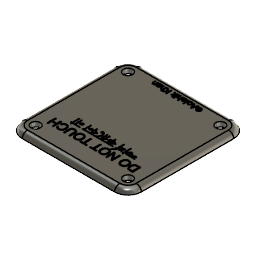
Sensor_Top (Autodesk Fusion 360 design; units mm, degrees)
part number: 2026-02-07-13-48-56-829
Autodesk Fusion 360 part; units mm, degrees
(part 1 of 2)
sketch "Sketch1" plane through (0, 0, 0) normal (0, 0, 1) x (1, 0, 0)
  line L0 (64.1962, 5) -> (20.1962, 5)
  line L1 (20.1962, 5) -> (20.1962, 49)
  line L2 (20.1962, 49) -> (64.1962, 49)
  line L3 (64.1962, 49) -> (64.1962, 5)
  circle A0 centre (59.1962, 10) radius 1.7
  circle A1 centre (25.1962, 10) radius 1.7
  circle A2 centre (59.1962, 44) radius 1.7
  circle A3 centre (25.1962, 44) radius 1.7
  dimension "d1" = 44
  dimension "d2" = 44
  dimension "d3" = 3.4
  dimension "d4" = 3.4
  dimension "d5" = 3.4
  dimension "d6" = 3.4
  dimension "d7" = 5
  dimension "d8" = 5
  dimension "d9" = 5
  dimension "d10" = 5
  dimension "d11" = 5
  dimension "d12" = 5
  dimension "d13" = 5
  dimension "d14" = 5
  constraint horizontal L0
  constraint vertical L1
  constraint horizontal L2
  constraint vertical L3
  measures "d1" distance of L0.start L0.end
  measures "d2" distance of L0.start L2.end
  measures "d3" diameter of A0
  measures "d4" diameter of A1
  measures "d5" diameter of A2
  measures "d6" diameter of A3
  measures "d7" distance of L3 A2.centre
  measures "d8" distance of L2 A2.centre
  measures "d9" distance of L2 A3.centre
  measures "d10" distance of L1 A3.centre
  measures "d11" distance of L1 A1.centre
  measures "d12" distance of L0 A1.centre
  measures "d13" distance of L0 A0.centre
  measures "d14" distance of L3 A0.centre
extrude "Extrude1" add sketch "Sketch1" along normal blind 1.75
sketch "Sketch2" plane through (0, 0, 1.75) normal (0, 0, 1) x (1, 0, 0)
  line L0 (57.9977, 15.8736) -> (57.9932, 12.8736)
  line L1 (57.9932, 12.8736) -> (56.9598, 12.8752)
  spline S0 degree 2 poles (56.9598, 12.8752) (56.6098, 12.8757) (56.4257, 12.9189) knots 0 0 0 1 1 1
  spline S1 degree 2 poles (56.4257, 12.9189) (56.168, 12.9787) (55.9861, 13.1345) knots 0 0 0 1 1 1
  spline S2 degree 2 poles (55.9861, 13.1345) (55.749, 13.3354) (55.6318, 13.6476) knots 0 0 0 1 1 1
  spline S3 degree 2 poles (55.6318, 13.6476) (55.5146, 13.9599) (55.5152, 14.361) knots 0 0 0 1 1 1
  spline S4 degree 2 poles (55.5152, 14.361) (55.5157, 14.7027) (55.5959, 14.9666) knots 0 0 0 1 1 1
  spline S5 degree 2 poles (55.5959, 14.9666) (55.6761, 15.2304) (55.8012, 15.4032) knots 0 0 0 1 1 1
  spline S6 degree 2 poles (55.8012, 15.4032) (55.9263, 15.5759) (56.0748, 15.6749) knots 0 0 0 1 1 1
  spline S7 degree 2 poles (56.0748, 15.6749) (56.2233, 15.7739) (56.4332, 15.8248) knots 0 0 0 1 1 1
  spline S8 degree 2 poles (56.4332, 15.8248) (56.643, 15.8756) (56.9152, 15.8752) knots 0 0 0 1 1 1
  line L2 (56.9152, 15.8752) -> (57.9977, 15.8736)
  line L3 (57.6002, 15.5202) -> (56.9596, 15.5211)
  spline S9 degree 2 poles (56.9596, 15.5211) (56.6629, 15.5216) (56.494, 15.4666) knots 0 0 0 1 1 1
  spline S10 degree 2 poles (56.494, 15.4666) (56.3251, 15.4116) (56.2247, 15.3115) knots 0 0 0 1 1 1
  spline S11 degree 2 poles (56.2247, 15.3115) (56.0833, 15.1705) (56.0041, 14.9322) knots 0 0 0 1 1 1
  spline S12 degree 2 poles (56.0041, 14.9322) (55.925, 14.6939) (55.9245, 14.3542) knots 0 0 0 1 1 1
  spline S13 degree 2 poles (55.9245, 14.3542) (55.9238, 13.8835) (56.0779, 13.6306) knots 0 0 0 1 1 1
  spline S14 degree 2 poles (56.0779, 13.6306) (56.232, 13.3776) (56.4529, 13.2913) knots 0 0 0 1 1 1
  spline S15 degree 2 poles (56.4529, 13.2913) (56.6124, 13.2297) (56.9664, 13.2292) knots 0 0 0 1 1 1
  line L4 (56.9664, 13.2292) -> (57.5967, 13.2282)
  line L5 (57.5967, 13.2282) -> (57.6002, 15.5202)
  spline S16 degree 2 poles (55.0896, 14.4168) (55.0885, 13.6699) (54.6868, 13.2479) knots 0 0 0 1 1 1
  spline S17 degree 2 poles (54.6868, 13.2479) (54.2851, 12.826) (53.6507, 12.8269) knots 0 0 0 1 1 1
  spline S18 degree 2 poles (53.6507, 12.8269) (53.2353, 12.8275) (52.902, 13.0265) knots 0 0 0 1 1 1
  spline S19 degree 2 poles (52.902, 13.0265) (52.5687, 13.2255) (52.3943, 13.5808) knots 0 0 0 1 1 1
  spline S20 degree 2 poles (52.3943, 13.5808) (52.2199, 13.9362) (52.2206, 14.3864) knots 0 0 0 1 1 1
  spline S21 degree 2 poles (52.2206, 14.3864) (52.2212, 14.8427) (52.406, 15.2026) knots 0 0 0 1 1 1
  spline S22 degree 2 poles (52.406, 15.2026) (52.5907, 15.5625) (52.9286, 15.7472) knots 0 0 0 1 1 1
  spline S23 degree 2 poles (52.9286, 15.7472) (53.2665, 15.9319) (53.6574, 15.9313) knots 0 0 0 1 1 1
  spline S24 degree 2 poles (53.6574, 15.9313) (54.081, 15.9306) (54.4142, 15.7255) knots 0 0 0 1 1 1
  spline S25 degree 2 poles (54.4142, 15.7255) (54.7475, 15.5204) (54.9189, 15.1661) knots 0 0 0 1 1 1
  spline S26 degree 2 poles (54.9189, 15.1661) (55.0902, 14.8118) (55.0896, 14.4168) knots 0 0 0 1 1 1
  spline S27 degree 2 poles (54.6804, 14.4236) (54.6812, 14.9659) (54.39, 15.2784) knots 0 0 0 1 1 1
  spline S28 degree 2 poles (54.39, 15.2784) (54.0989, 15.5909) (53.6589, 15.5916) knots 0 0 0 1 1 1
  spline S29 degree 2 poles (53.6589, 15.5916) (53.2108, 15.5922) (52.9207, 15.2775) knots 0 0 0 1 1 1
  spline S30 degree 2 poles (52.9207, 15.2775) (52.6307, 14.9628) (52.6298, 14.3837) knots 0 0 0 1 1 1
  spline S31 degree 2 poles (52.6298, 14.3837) (52.6293, 14.0174) (52.7527, 13.744) knots 0 0 0 1 1 1
  spline S32 degree 2 poles (52.7527, 13.744) (52.8761, 13.4706) (53.1143, 13.3199) knots 0 0 0 1 1 1
  spline S33 degree 2 poles (53.1143, 13.3199) (53.3524, 13.1691) (53.6492, 13.1687) knots 0 0 0 1 1 1
  spline S34 degree 2 poles (53.6492, 13.1687) (54.0707, 13.168) (54.375, 13.4571) knots 0 0 0 1 1 1
  spline S35 degree 2 poles (54.375, 13.4571) (54.6794, 13.7462) (54.6804, 14.4236) knots 0 0 0 1 1 1
  line L6 (50.5509, 15.8848) -> (50.5464, 12.8848)
  line L7 (50.5464, 12.8848) -> (50.1392, 12.8854)
  line L8 (50.1392, 12.8854) -> (48.567, 15.2431)
  line L9 (48.567, 15.2431) -> (48.5635, 12.8878)
  line L10 (48.5635, 12.8878) -> (48.1828, 12.8883)
  line L11 (48.1828, 12.8883) -> (48.1873, 15.8883)
  line L12 (48.1873, 15.8883) -> (48.5946, 15.8877)
  line L13 (48.5946, 15.8877) -> (50.1667, 13.5279)
  line L14 (50.1667, 13.5279) -> (50.1703, 15.8853)
  line L15 (50.1703, 15.8853) -> (50.5509, 15.8848)
  spline S36 degree 2 poles (47.6388, 14.428) (47.6376, 13.6811) (47.2359, 13.2591) knots 0 0 0 1 1 1
  spline S37 degree 2 poles (47.2359, 13.2591) (46.8342, 12.8371) (46.1998, 12.8381) knots 0 0 0 1 1 1
  spline S38 degree 2 poles (46.1998, 12.8381) (45.7844, 12.8387) (45.4511, 13.0377) knots 0 0 0 1 1 1
  spline S39 degree 2 poles (45.4511, 13.0377) (45.1179, 13.2367) (44.9434, 13.592) knots 0 0 0 1 1 1
  spline S40 degree 2 poles (44.9434, 13.592) (44.769, 13.9473) (44.7697, 14.3975) knots 0 0 0 1 1 1
  spline S41 degree 2 poles (44.7697, 14.3975) (44.7704, 14.8539) (44.9551, 15.2138) knots 0 0 0 1 1 1
  spline S42 degree 2 poles (44.9551, 15.2138) (45.1398, 15.5737) (45.4777, 15.7583) knots 0 0 0 1 1 1
  spline S43 degree 2 poles (45.4777, 15.7583) (45.8157, 15.943) (46.2065, 15.9425) knots 0 0 0 1 1 1
  spline S44 degree 2 poles (46.2065, 15.9425) (46.6301, 15.9418) (46.9634, 15.7367) knots 0 0 0 1 1 1
  spline S45 degree 2 poles (46.9634, 15.7367) (47.2966, 15.5315) (47.468, 15.1773) knots 0 0 0 1 1 1
  spline S46 degree 2 poles (47.468, 15.1773) (47.6394, 14.823) (47.6388, 14.428) knots 0 0 0 1 1 1
  spline S47 degree 2 poles (47.2295, 14.4348) (47.2303, 14.9771) (46.9392, 15.2896) knots 0 0 0 1 1 1
  spline S48 degree 2 poles (46.9392, 15.2896) (46.648, 15.6021) (46.2081, 15.6027) knots 0 0 0 1 1 1
  spline S49 degree 2 poles (46.2081, 15.6027) (45.7599, 15.6034) (45.4699, 15.2887) knots 0 0 0 1 1 1
  spline S50 degree 2 poles (45.4699, 15.2887) (45.1798, 14.974) (45.179, 14.3949) knots 0 0 0 1 1 1
  spline S51 degree 2 poles (45.179, 14.3949) (45.1784, 14.0286) (45.3018, 13.7552) knots 0 0 0 1 1 1
  spline S52 degree 2 poles (45.3018, 13.7552) (45.4252, 13.4818) (45.6634, 13.3311) knots 0 0 0 1 1 1
  spline S53 degree 2 poles (45.6634, 13.3311) (45.9016, 13.1803) (46.1983, 13.1798) knots 0 0 0 1 1 1
  spline S54 degree 2 poles (46.1983, 13.1798) (46.6198, 13.1792) (46.9242, 13.4683) knots 0 0 0 1 1 1
  spline S55 degree 2 poles (46.9242, 13.4683) (47.2285, 13.7574) (47.2295, 14.4348) knots 0 0 0 1 1 1
  line L16 (43.497, 15.8954) -> (43.4931, 13.2494)
  line L17 (43.4931, 13.2494) -> (44.4815, 13.2479)
  line L18 (44.4815, 13.2479) -> (44.4809, 12.8939)
  line L19 (44.4809, 12.8939) -> (42.103, 12.8974)
  line L20 (42.103, 12.8974) -> (42.1036, 13.2515)
  line L21 (42.1036, 13.2515) -> (43.0961, 13.25)
  line L22 (43.0961, 13.25) -> (43.1, 15.896)
  line L23 (43.1, 15.896) -> (43.497, 15.8954)
  line L24 (39.924, 15.9007) -> (39.9201, 13.2547)
  line L25 (39.9201, 13.2547) -> (40.9085, 13.2533)
  line L26 (40.9085, 13.2533) -> (40.9079, 12.8992)
  line L27 (40.9079, 12.8992) -> (38.53, 12.9028)
  line L28 (38.53, 12.9028) -> (38.5306, 13.2568)
  line L29 (38.5306, 13.2568) -> (39.5231, 13.2553)
  line L30 (39.5231, 13.2553) -> (39.527, 15.9013)
  line L31 (39.527, 15.9013) -> (39.924, 15.9007)
  spline S56 degree 2 poles (38.3216, 14.442) (38.3205, 13.6951) (37.9187, 13.2731) knots 0 0 0 1 1 1
  spline S57 degree 2 poles (37.9187, 13.2731) (37.517, 12.8511) (36.8826, 12.8521) knots 0 0 0 1 1 1
  spline S58 degree 2 poles (36.8826, 12.8521) (36.4672, 12.8527) (36.134, 13.0517) knots 0 0 0 1 1 1
  spline S59 degree 2 poles (36.134, 13.0517) (35.8007, 13.2507) (35.6263, 13.606) knots 0 0 0 1 1 1
  spline S60 degree 2 poles (35.6263, 13.606) (35.4518, 13.9613) (35.4525, 14.4115) knots 0 0 0 1 1 1
  spline S61 degree 2 poles (35.4525, 14.4115) (35.4532, 14.8679) (35.6379, 15.2277) knots 0 0 0 1 1 1
  spline S62 degree 2 poles (35.6379, 15.2277) (35.8226, 15.5876) (36.1605, 15.7723) knots 0 0 0 1 1 1
  spline S63 degree 2 poles (36.1605, 15.7723) (36.4985, 15.957) (36.8893, 15.9564) knots 0 0 0 1 1 1
  spline S64 degree 2 poles (36.8893, 15.9564) (37.3129, 15.9558) (37.6462, 15.7507) knots 0 0 0 1 1 1
  spline S65 degree 2 poles (37.6462, 15.7507) (37.9794, 15.5455) (38.1508, 15.1912) knots 0 0 0 1 1 1
  spline S66 degree 2 poles (38.1508, 15.1912) (38.3222, 14.837) (38.3216, 14.442) knots 0 0 0 1 1 1
  spline S67 degree 2 poles (37.9123, 14.4488) (37.9131, 14.991) (37.622, 15.3036) knots 0 0 0 1 1 1
  spline S68 degree 2 poles (37.622, 15.3036) (37.3308, 15.6161) (36.8909, 15.6167) knots 0 0 0 1 1 1
  spline S69 degree 2 poles (36.8909, 15.6167) (36.4427, 15.6174) (36.1527, 15.3027) knots 0 0 0 1 1 1
  spline S70 degree 2 poles (36.1527, 15.3027) (35.8626, 14.988) (35.8618, 14.4089) knots 0 0 0 1 1 1
  spline S71 degree 2 poles (35.8618, 14.4089) (35.8612, 14.0426) (35.9846, 13.7692) knots 0 0 0 1 1 1
  spline S72 degree 2 poles (35.9846, 13.7692) (36.108, 13.4958) (36.3462, 13.345) knots 0 0 0 1 1 1
  spline S73 degree 2 poles (36.3462, 13.345) (36.5844, 13.1943) (36.8811, 13.1938) knots 0 0 0 1 1 1
  spline S74 degree 2 poles (36.8811, 13.1938) (37.3027, 13.1932) (37.607, 13.4823) knots 0 0 0 1 1 1
  spline S75 degree 2 poles (37.607, 13.4823) (37.9113, 13.7714) (37.9123, 14.4488) knots 0 0 0 1 1 1
  line L32 (32.97, 12.9111) -> (32.573, 12.9117)
  line L33 (32.573, 12.9117) -> (32.5756, 14.645)
  spline S76 degree 2 poles (32.5756, 14.645) (32.5763, 15.0973) (32.679, 15.3632) knots 0 0 0 1 1 1
  spline S77 degree 2 poles (32.679, 15.3632) (32.7817, 15.629) (33.049, 15.7954) knots 0 0 0 1 1 1
  spline S78 degree 2 poles (33.049, 15.7954) (33.3164, 15.9618) (33.7502, 15.9611) knots 0 0 0 1 1 1
  spline S79 degree 2 poles (33.7502, 15.9611) (34.1717, 15.9605) (34.4396, 15.8148) knots 0 0 0 1 1 1
  spline S80 degree 2 poles (34.4396, 15.8148) (34.7075, 15.6691) (34.8216, 15.3937) knots 0 0 0 1 1 1
  spline S81 degree 2 poles (34.8216, 15.3937) (34.9358, 15.1183) (34.9351, 14.6415) knots 0 0 0 1 1 1
  line L34 (34.9351, 14.6415) -> (34.9325, 12.9082)
  line L35 (34.9325, 12.9082) -> (34.5355, 12.9088)
  line L36 (34.5355, 12.9088) -> (34.5381, 14.64)
  spline S82 degree 2 poles (34.5381, 14.64) (34.5387, 15.0309) (34.4663, 15.2162) knots 0 0 0 1 1 1
  spline S83 degree 2 poles (34.4663, 15.2162) (34.394, 15.4015) (34.2171, 15.502) knots 0 0 0 1 1 1
  spline S84 degree 2 poles (34.2171, 15.502) (34.0402, 15.6026) (33.7844, 15.603) knots 0 0 0 1 1 1
  spline S85 degree 2 poles (33.7844, 15.603) (33.3465, 15.6036) (33.16, 15.4054) knots 0 0 0 1 1 1
  spline S86 degree 2 poles (33.16, 15.4054) (32.9735, 15.2072) (32.9726, 14.6424) knots 0 0 0 1 1 1
  line L37 (32.9726, 14.6424) -> (32.97, 12.9111)
  line L38 (29.7745, 14.8641) -> (29.3776, 14.965)
  spline S87 degree 2 poles (29.3776, 14.965) (29.5032, 15.4539) (29.8279, 15.7102) knots 0 0 0 1 1 1
  spline S88 degree 2 poles (29.8279, 15.7102) (30.1526, 15.9665) (30.6213, 15.9658) knots 0 0 0 1 1 1
  spline S89 degree 2 poles (30.6213, 15.9658) (31.1063, 15.9651) (31.4099, 15.7672) knots 0 0 0 1 1 1
  spline S90 degree 2 poles (31.4099, 15.7672) (31.7134, 15.5692) (31.8715, 15.1945) knots 0 0 0 1 1 1
  spline S91 degree 2 poles (31.8715, 15.1945) (32.0295, 14.8198) (32.0289, 14.3901) knots 0 0 0 1 1 1
  spline S92 degree 2 poles (32.0289, 14.3901) (32.0282, 13.9214) (31.8486, 13.5728) knots 0 0 0 1 1 1
  spline S93 degree 2 poles (31.8486, 13.5728) (31.669, 13.2242) (31.3382, 13.0435) knots 0 0 0 1 1 1
  spline S94 degree 2 poles (31.3382, 13.0435) (31.0075, 12.8629) (30.6105, 12.8635) knots 0 0 0 1 1 1
  spline S95 degree 2 poles (30.6105, 12.8635) (30.1603, 12.8642) (29.8537, 13.0939) knots 0 0 0 1 1 1
  spline S96 degree 2 poles (29.8537, 13.0939) (29.547, 13.3235) (29.4269, 13.7391) knots 0 0 0 1 1 1
  line L39 (29.4269, 13.7391) -> (29.8179, 13.8306)
  spline S97 degree 2 poles (29.8179, 13.8306) (29.9218, 13.503) (30.1201, 13.3534) knots 0 0 0 1 1 1
  spline S98 degree 2 poles (30.1201, 13.3534) (30.3183, 13.2037) (30.6192, 13.2032) knots 0 0 0 1 1 1
  spline S99 degree 2 poles (30.6192, 13.2032) (30.965, 13.2027) (31.1975, 13.3681) knots 0 0 0 1 1 1
  spline S100 degree 2 poles (31.1975, 13.3681) (31.43, 13.5335) (31.5246, 13.8127) knots 0 0 0 1 1 1
  spline S101 degree 2 poles (31.5246, 13.8127) (31.6191, 14.0919) (31.6196, 14.3886) knots 0 0 0 1 1 1
  spline S102 degree 2 poles (31.6196, 14.3886) (31.6202, 14.7713) (31.5091, 15.0569) knots 0 0 0 1 1 1
  spline S103 degree 2 poles (31.5091, 15.0569) (31.398, 15.3426) (31.1628, 15.4841) knots 0 0 0 1 1 1
  spline S104 degree 2 poles (31.1628, 15.4841) (30.9277, 15.6257) (30.6535, 15.6261) knots 0 0 0 1 1 1
  spline S105 degree 2 poles (30.6535, 15.6261) (30.3199, 15.6266) (30.0884, 15.4346) knots 0 0 0 1 1 1
  spline S106 degree 2 poles (30.0884, 15.4346) (29.8569, 15.2426) (29.7745, 14.8641) knots 0 0 0 1 1 1
  line L40 (28.8777, 15.9173) -> (28.8732, 12.9173)
  line L41 (28.8732, 12.9173) -> (28.4762, 12.9179)
  line L42 (28.4762, 12.9179) -> (28.478, 14.1498)
  line L43 (28.478, 14.1498) -> (26.9187, 14.1522)
  line L44 (26.9187, 14.1522) -> (26.9168, 12.9202)
  line L45 (26.9168, 12.9202) -> (26.5198, 12.9208)
  line L46 (26.5198, 12.9208) -> (26.5243, 15.9208)
  line L47 (26.5243, 15.9208) -> (26.9213, 15.9202)
  line L48 (26.9213, 15.9202) -> (26.9192, 14.5062)
  line L49 (26.9192, 14.5062) -> (28.4786, 14.5038)
  line L50 (28.4786, 14.5038) -> (28.4807, 15.9179)
  line L51 (28.4807, 15.9179) -> (28.8777, 15.9173)
  line L52 (49.5473, 17.5944) -> (50.0835, 17.5936)
  line L53 (50.0835, 17.5936) -> (50.0876, 20.3111)
  line L54 (50.0876, 20.3111) -> (50.2965, 20.1068)
  line L55 (50.2965, 20.1068) -> (50.2942, 18.6003)
  spline S107 degree 2 poles (50.2942, 18.6003) (50.2941, 18.5506) (50.3137, 18.4878) knots 0 0 0 1 1 1
  spline S108 degree 2 poles (50.3137, 18.4878) (50.3332, 18.425) (50.3645, 18.3634) knots 0 0 0 1 1 1
  spline S109 degree 2 poles (50.3645, 18.3634) (50.3958, 18.3019) (50.431, 18.2456) knots 0 0 0 1 1 1
  spline S110 degree 2 poles (50.431, 18.2456) (50.4662, 18.1894) (50.4975, 18.1501) knots 0 0 0 1 1 1
  line L56 (50.4975, 18.1501) -> (51.5662, 19.1738)
  line L57 (51.5662, 19.1738) -> (51.8798, 19.0059)
  spline S111 degree 2 poles (51.8798, 19.0059) (51.6493, 18.7865) (51.5393, 18.6703) knots 0 0 0 1 1 1
  spline S112 degree 2 poles (51.5393, 18.6703) (51.4293, 18.5541) (51.4292, 18.5148) knots 0 0 0 1 1 1
  spline S113 degree 2 poles (51.4292, 18.5148) (51.4291, 18.4259) (51.497, 18.3761) knots 0 0 0 1 1 1
  spline S114 degree 2 poles (51.497, 18.3761) (51.5649, 18.3263) (51.6539, 18.3262) knots 0 0 0 1 1 1
  spline S115 degree 2 poles (51.6539, 18.3262) (51.7428, 18.3261) (51.8292, 18.3586) knots 0 0 0 1 1 1
  spline S116 degree 2 poles (51.8292, 18.3586) (51.9155, 18.3912) (52.0032, 18.4303) knots 0 0 0 1 1 1
  spline S117 degree 2 poles (52.0032, 18.4303) (52.0909, 18.4694) (52.1786, 18.5019) knots 0 0 0 1 1 1
  spline S118 degree 2 poles (52.1786, 18.5019) (52.2662, 18.5345) (52.3578, 18.5344) knots 0 0 0 1 1 1
  spline S119 degree 2 poles (52.3578, 18.5344) (52.4912, 18.5342) (52.6048, 18.4791) knots 0 0 0 1 1 1
  spline S120 degree 2 poles (52.6048, 18.4791) (52.7185, 18.424) (52.8073, 18.331) knots 0 0 0 1 1 1
  spline S121 degree 2 poles (52.8073, 18.331) (52.8961, 18.238) (52.9587, 18.1189) knots 0 0 0 1 1 1
  spline S122 degree 2 poles (52.9587, 18.1189) (53.0213, 17.9998) (53.0499, 17.8742) knots 0 0 0 1 1 1
  spline S123 degree 2 poles (53.0499, 17.8742) (53.1626, 18.0519) (53.2374, 18.1943) knots 0 0 0 1 1 1
  spline S124 degree 2 poles (53.2374, 18.1943) (53.3121, 18.3368) (53.3672, 18.4361) knots 0 0 0 1 1 1
  spline S125 degree 2 poles (53.3672, 18.4361) (53.4223, 18.5354) (53.4681, 18.5876) knots 0 0 0 1 1 1
  spline S126 degree 2 poles (53.4681, 18.5876) (53.514, 18.6399) (53.5689, 18.6398) knots 0 0 0 1 1 1
  spline S127 degree 2 poles (53.5689, 18.6398) (53.6108, 18.6397) (53.6656, 18.6161) knots 0 0 0 1 1 1
  spline S128 degree 2 poles (53.6656, 18.6161) (53.7205, 18.5925) (53.7845, 18.5374) knots 0 0 0 1 1 1
  spline S129 degree 2 poles (53.7845, 18.5374) (53.8485, 18.4824) (53.9203, 18.3908) knots 0 0 0 1 1 1
  spline S130 degree 2 poles (53.9203, 18.3908) (53.9921, 18.2991) (54.0678, 18.163) knots 0 0 0 1 1 1
  line L58 (54.0678, 18.163) -> (53.9395, 18.0821)
  spline S131 degree 2 poles (53.9395, 18.0821) (53.9212, 18.1214) (53.8964, 18.1619) knots 0 0 0 1 1 1
  spline S132 degree 2 poles (53.8964, 18.1619) (53.8717, 18.2025) (53.8429, 18.2353) knots 0 0 0 1 1 1
  spline S133 degree 2 poles (53.8429, 18.2353) (53.8142, 18.268) (53.7855, 18.2903) knots 0 0 0 1 1 1
  spline S134 degree 2 poles (53.7855, 18.2903) (53.7567, 18.3126) (53.7306, 18.3126) knots 0 0 0 1 1 1
  spline S135 degree 2 poles (53.7306, 18.3126) (53.6573, 18.3127) (53.6075, 18.2448) knots 0 0 0 1 1 1
  spline S136 degree 2 poles (53.6075, 18.2448) (53.5577, 18.1768) (53.5053, 18.071) knots 0 0 0 1 1 1
  spline S137 degree 2 poles (53.5053, 18.071) (53.4528, 17.9651) (53.3833, 17.8371) knots 0 0 0 1 1 1
  spline S138 degree 2 poles (53.3833, 17.8371) (53.3138, 17.709) (53.1985, 17.5889) knots 0 0 0 1 1 1
  line L59 (53.1985, 17.5889) -> (54.1323, 17.5875)
  line L60 (54.1323, 17.5875) -> (54.2758, 17.3911)
  line L61 (54.2758, 17.3911) -> (52.1573, 17.3943)
  line L62 (52.1573, 17.3943) -> (52.0242, 17.5907)
  line L63 (52.0242, 17.5907) -> (52.0059, 17.6221)
  spline S139 degree 2 poles (52.0059, 17.6221) (51.8776, 17.5229) (51.7232, 17.4617) knots 0 0 0 1 1 1
  spline S140 degree 2 poles (51.7232, 17.4617) (51.5688, 17.4004) (51.3962, 17.4007) knots 0 0 0 1 1 1
  spline S141 degree 2 poles (51.3962, 17.4007) (51.1948, 17.401) (51.0314, 17.4588) knots 0 0 0 1 1 1
  spline S142 degree 2 poles (51.0314, 17.4588) (50.868, 17.5166) (50.7348, 17.6175) knots 0 0 0 1 1 1
  spline S143 degree 2 poles (50.7348, 17.6175) (50.6015, 17.7184) (50.4932, 17.8545) knots 0 0 0 1 1 1
  spline S144 degree 2 poles (50.4932, 17.8545) (50.3848, 17.9907) (50.2935, 18.1478) knots 0 0 0 1 1 1
  line L64 (50.2935, 18.1478) -> (50.2916, 16.8871)
  spline S145 degree 2 poles (50.2916, 16.8871) (50.242, 16.9107) (50.2094, 16.9761) knots 0 0 0 1 1 1
  spline S146 degree 2 poles (50.2094, 16.9761) (50.1768, 17.0416) (50.1547, 17.1201) knots 0 0 0 1 1 1
  spline S147 degree 2 poles (50.1547, 17.1201) (50.1326, 17.1986) (50.117, 17.2745) knots 0 0 0 1 1 1
  spline S148 degree 2 poles (50.117, 17.2745) (50.1014, 17.3503) (50.0858, 17.3974) knots 0 0 0 1 1 1
  line L65 (50.0858, 17.3974) -> (49.6908, 17.398)
  line L66 (49.6908, 17.398) -> (49.5473, 17.5944)
  spline S149 degree 2 poles (52.09, 17.8914) (52.0899, 17.8103) (52.1225, 17.7475) knots 0 0 0 1 1 1
  spline S150 degree 2 poles (52.1225, 17.7475) (52.1551, 17.6846) (52.2229, 17.5904) knots 0 0 0 1 1 1
  line L67 (52.2229, 17.5904) -> (52.903, 17.5893)
  spline S151 degree 2 poles (52.903, 17.5893) (52.9448, 17.5893) (52.954, 17.6298) knots 0 0 0 1 1 1
  spline S152 degree 2 poles (52.954, 17.6298) (52.9633, 17.6703) (52.9633, 17.7148) knots 0 0 0 1 1 1
  spline S153 degree 2 poles (52.9633, 17.7148) (52.9635, 17.7985) (52.9165, 17.8901) knots 0 0 0 1 1 1
  spline S154 degree 2 poles (52.9165, 17.8901) (52.8696, 17.9817) (52.7925, 18.0577) knots 0 0 0 1 1 1
  spline S155 degree 2 poles (52.7925, 18.0577) (52.7155, 18.1337) (52.6149, 18.1835) knots 0 0 0 1 1 1
  spline S156 degree 2 poles (52.6149, 18.1835) (52.5142, 18.2333) (52.407, 18.2335) knots 0 0 0 1 1 1
  spline S157 degree 2 poles (52.407, 18.2335) (52.3442, 18.2336) (52.2867, 18.2102) knots 0 0 0 1 1 1
  spline S158 degree 2 poles (52.2867, 18.2102) (52.2291, 18.1867) (52.1859, 18.141) knots 0 0 0 1 1 1
  spline S159 degree 2 poles (52.1859, 18.141) (52.1426, 18.0953) (52.1164, 18.0326) knots 0 0 0 1 1 1
  spline S160 degree 2 poles (52.1164, 18.0326) (52.0901, 17.9698) (52.09, 17.8914) knots 0 0 0 1 1 1
  spline S161 degree 2 poles (50.7482, 17.8829) (50.8736, 17.7833) (51.0226, 17.7334) knots 0 0 0 1 1 1
  spline S162 degree 2 poles (51.0226, 17.7334) (51.1716, 17.6835) (51.3286, 17.6833) knots 0 0 0 1 1 1
  spline S163 degree 2 poles (51.3286, 17.6833) (51.4724, 17.683) (51.619, 17.7391) knots 0 0 0 1 1 1
  spline S164 degree 2 poles (51.619, 17.7391) (51.7655, 17.7951) (51.8913, 17.9466) knots 0 0 0 1 1 1
  spline S165 degree 2 poles (51.8913, 17.9466) (51.8861, 17.9754) (51.8836, 18.0041) knots 0 0 0 1 1 1
  spline S166 degree 2 poles (51.8836, 18.0041) (51.881, 18.0329) (51.881, 18.0591) knots 0 0 0 1 1 1
  spline S167 degree 2 poles (51.881, 18.0591) (51.881, 18.0748) (51.8824, 18.0918) knots 0 0 0 1 1 1
  spline S168 degree 2 poles (51.8824, 18.0918) (51.8837, 18.1088) (51.8864, 18.1244) knots 0 0 0 1 1 1
  spline S169 degree 2 poles (51.8864, 18.1244) (51.8392, 18.1088) (51.7895, 18.0971) knots 0 0 0 1 1 1
  spline S170 degree 2 poles (51.7895, 18.0971) (51.7398, 18.0854) (51.6875, 18.0855) knots 0 0 0 1 1 1
  spline S171 degree 2 poles (51.6875, 18.0855) (51.562, 18.0857) (51.4562, 18.1643) knots 0 0 0 1 1 1
  spline S172 degree 2 poles (51.4562, 18.1643) (51.3503, 18.243) (51.2904, 18.4078) knots 0 0 0 1 1 1
  line L68 (51.2904, 18.4078) -> (50.7482, 17.8829)
  line L69 (46.9527, 17.5983) -> (47.4889, 17.5975)
  line L70 (47.4889, 17.5975) -> (47.493, 20.3046)
  line L71 (47.493, 20.3046) -> (47.7019, 20.095)
  line L72 (47.7019, 20.095) -> (47.6993, 18.4028)
  spline S173 degree 2 poles (47.6993, 18.4028) (47.6993, 18.374) (47.7214, 18.3125) knots 0 0 0 1 1 1
  spline S174 degree 2 poles (47.7214, 18.3125) (47.7436, 18.251) (47.7827, 18.1764) knots 0 0 0 1 1 1
  spline S175 degree 2 poles (47.7827, 18.1764) (47.8218, 18.1018) (47.8753, 18.0206) knots 0 0 0 1 1 1
  spline S176 degree 2 poles (47.8753, 18.0206) (47.9288, 17.9395) (47.9888, 17.874) knots 0 0 0 1 1 1
  spline S177 degree 2 poles (47.9888, 17.874) (48.0489, 17.8085) (48.1168, 17.7653) knots 0 0 0 1 1 1
  spline S178 degree 2 poles (48.1168, 17.7653) (48.1848, 17.722) (48.2502, 17.7219) knots 0 0 0 1 1 1
  spline S179 degree 2 poles (48.2502, 17.7219) (48.3077, 17.7218) (48.3522, 17.7453) knots 0 0 0 1 1 1
  spline S180 degree 2 poles (48.3522, 17.7453) (48.3967, 17.7688) (48.4321, 17.8053) knots 0 0 0 1 1 1
  spline S181 degree 2 poles (48.4321, 17.8053) (48.4674, 17.8419) (48.4976, 17.8902) knots 0 0 0 1 1 1
  spline S182 degree 2 poles (48.4976, 17.8902) (48.5277, 17.9386) (48.5566, 17.9882) knots 0 0 0 1 1 1
  spline S183 degree 2 poles (48.5566, 17.9882) (48.3267, 18.1612) (48.2066, 18.334) knots 0 0 0 1 1 1
  spline S184 degree 2 poles (48.2066, 18.334) (48.0866, 18.5068) (48.0868, 18.6481) knots 0 0 0 1 1 1
  spline S185 degree 2 poles (48.0868, 18.6481) (48.087, 18.7657) (48.1577, 18.8402) knots 0 0 0 1 1 1
  spline S186 degree 2 poles (48.1577, 18.8402) (48.2284, 18.9146) (48.3383, 18.9145) knots 0 0 0 1 1 1
  spline S187 degree 2 poles (48.3383, 18.9145) (48.4063, 18.9144) (48.4716, 18.8868) knots 0 0 0 1 1 1
  spline S188 degree 2 poles (48.4716, 18.8868) (48.537, 18.8592) (48.5918, 18.8134) knots 0 0 0 1 1 1
  spline S189 degree 2 poles (48.5918, 18.8134) (48.6467, 18.7675) (48.6845, 18.7073) knots 0 0 0 1 1 1
  spline S190 degree 2 poles (48.6845, 18.7073) (48.7224, 18.6471) (48.7353, 18.5817) knots 0 0 0 1 1 1
  spline S191 degree 2 poles (48.7353, 18.5817) (48.7694, 18.6444) (48.8166, 18.7071) knots 0 0 0 1 1 1
  spline S192 degree 2 poles (48.8166, 18.7071) (48.8638, 18.7698) (48.9201, 18.8207) knots 0 0 0 1 1 1
  spline S193 degree 2 poles (48.9201, 18.8207) (48.9764, 18.8716) (49.0379, 18.9029) knots 0 0 0 1 1 1
  spline S194 degree 2 poles (49.0379, 18.9029) (49.0994, 18.9342) (49.1622, 18.9341) knots 0 0 0 1 1 1
  spline S195 degree 2 poles (49.1622, 18.9341) (49.3034, 18.9339) (49.3805, 18.8671) knots 0 0 0 1 1 1
  spline S196 degree 2 poles (49.3805, 18.8671) (49.4576, 18.8003) (49.4573, 18.6355) knots 0 0 0 1 1 1
  spline S197 degree 2 poles (49.4573, 18.6355) (49.4572, 18.5387) (49.4073, 18.4407) knots 0 0 0 1 1 1
  spline S198 degree 2 poles (49.4073, 18.4407) (49.3575, 18.3427) (49.2841, 18.2591) knots 0 0 0 1 1 1
  spline S199 degree 2 poles (49.2841, 18.2591) (49.2108, 18.1756) (49.1283, 18.1103) knots 0 0 0 1 1 1
  spline S200 degree 2 poles (49.1283, 18.1103) (49.0458, 18.045) (48.9803, 18.0137) knots 0 0 0 1 1 1
  spline S201 degree 2 poles (48.9803, 18.0137) (49.0038, 17.9379) (49.0429, 17.8633) knots 0 0 0 1 1 1
  spline S202 degree 2 poles (49.0429, 17.8633) (49.082, 17.7887) (49.1368, 17.7284) knots 0 0 0 1 1 1
  spline S203 degree 2 poles (49.1368, 17.7284) (49.1917, 17.6682) (49.2622, 17.6315) knots 0 0 0 1 1 1
  spline S204 degree 2 poles (49.2622, 17.6315) (49.3328, 17.5947) (49.4191, 17.5946) knots 0 0 0 1 1 1
  line L73 (49.4191, 17.5946) -> (49.7304, 17.5941)
  line L74 (49.7304, 17.5941) -> (49.8739, 17.3977)
  line L75 (49.8739, 17.3977) -> (49.3639, 17.3985)
  spline S205 degree 2 poles (49.3639, 17.3985) (49.2828, 17.3986) (49.2031, 17.4419) knots 0 0 0 1 1 1
  spline S206 degree 2 poles (49.2031, 17.4419) (49.1234, 17.4852) (49.0581, 17.5533) knots 0 0 0 1 1 1
  spline S207 degree 2 poles (49.0581, 17.5533) (48.9928, 17.6214) (48.9485, 17.7078) knots 0 0 0 1 1 1
  spline S208 degree 2 poles (48.9485, 17.7078) (48.9042, 17.7942) (48.8938, 17.8805) knots 0 0 0 1 1 1
  spline S209 degree 2 poles (48.8938, 17.8805) (48.7208, 17.627) (48.5833, 17.5109) knots 0 0 0 1 1 1
  spline S210 degree 2 poles (48.5833, 17.5109) (48.4458, 17.3947) (48.3621, 17.3948) knots 0 0 0 1 1 1
  spline S211 degree 2 poles (48.3621, 17.3948) (48.2575, 17.395) (48.1595, 17.4566) knots 0 0 0 1 1 1
  spline S212 degree 2 poles (48.1595, 17.4566) (48.0615, 17.5182) (47.9754, 17.6099) knots 0 0 0 1 1 1
  spline S213 degree 2 poles (47.9754, 17.6099) (47.8892, 17.7015) (47.8187, 17.8089) knots 0 0 0 1 1 1
  spline S214 degree 2 poles (47.8187, 17.8089) (47.7483, 17.9162) (47.6987, 18.0052) knots 0 0 0 1 1 1
  line L76 (47.6987, 18.0052) -> (47.697, 16.891)
  spline S215 degree 2 poles (47.697, 16.891) (47.6474, 16.9146) (47.6148, 16.9801) knots 0 0 0 1 1 1
  spline S216 degree 2 poles (47.6148, 16.9801) (47.5822, 17.0455) (47.5601, 17.124) knots 0 0 0 1 1 1
  spline S217 degree 2 poles (47.5601, 17.124) (47.538, 17.2025) (47.5224, 17.2784) knots 0 0 0 1 1 1
  spline S218 degree 2 poles (47.5224, 17.2784) (47.5068, 17.3542) (47.4912, 17.4013) knots 0 0 0 1 1 1
  line L77 (47.4912, 17.4013) -> (47.0962, 17.4019)
  line L78 (47.0962, 17.4019) -> (46.9527, 17.5983)
  line L79 (46.485, 16.2076) -> (47.4386, 17.187)
  line L80 (47.4386, 17.187) -> (47.9172, 17.1862)
  line L81 (47.9172, 17.1862) -> (46.6786, 16.2073)
  line L82 (46.6786, 16.2073) -> (46.485, 16.2076)
  line L83 (42.8542, 17.6045) -> (44.3502, 17.6022)
  line L84 (44.3502, 17.6022) -> (44.3505, 17.7696)
  spline S219 degree 2 poles (44.3505, 17.7696) (44.1125, 17.8092) (43.9322, 17.9063) knots 0 0 0 1 1 1
  spline S220 degree 2 poles (43.9322, 17.9063) (43.7519, 18.0033) (43.6318, 18.1356) knots 0 0 0 1 1 1
  spline S221 degree 2 poles (43.6318, 18.1356) (43.5117, 18.2679) (43.4517, 18.4236) knots 0 0 0 1 1 1
  spline S222 degree 2 poles (43.4517, 18.4236) (43.3918, 18.5793) (43.3921, 18.7362) knots 0 0 0 1 1 1
  spline S223 degree 2 poles (43.3921, 18.7362) (43.3922, 18.8225) (43.4172, 18.9297) knots 0 0 0 1 1 1
  spline S224 degree 2 poles (43.4172, 18.9297) (43.4422, 19.0369) (43.4934, 19.1297) knots 0 0 0 1 1 1
  spline S225 degree 2 poles (43.4934, 19.1297) (43.5445, 19.2225) (43.6217, 19.2864) knots 0 0 0 1 1 1
  spline S226 degree 2 poles (43.6217, 19.2864) (43.699, 19.3504) (43.801, 19.3502) knots 0 0 0 1 1 1
  spline S227 degree 2 poles (43.801, 19.3502) (43.8559, 19.3502) (43.9069, 19.3318) knots 0 0 0 1 1 1
  spline S228 degree 2 poles (43.9069, 19.3318) (43.9579, 19.3134) (43.9971, 19.2767) knots 0 0 0 1 1 1
  spline S229 degree 2 poles (43.9971, 19.2767) (44.0362, 19.24) (44.061, 19.1877) knots 0 0 0 1 1 1
  spline S230 degree 2 poles (44.061, 19.1877) (44.0858, 19.1353) (44.0857, 19.0673) knots 0 0 0 1 1 1
  spline S231 degree 2 poles (44.0857, 19.0673) (44.0856, 19.0203) (44.0685, 18.9654) knots 0 0 0 1 1 1
  spline S232 degree 2 poles (44.0685, 18.9654) (44.0514, 18.9105) (44.0174, 18.8634) knots 0 0 0 1 1 1
  spline S233 degree 2 poles (44.0174, 18.8634) (43.9833, 18.8164) (43.9335, 18.7838) knots 0 0 0 1 1 1
  spline S234 degree 2 poles (43.9335, 18.7838) (43.8838, 18.7512) (43.8158, 18.7513) knots 0 0 0 1 1 1
  spline S235 degree 2 poles (43.8158, 18.7513) (43.7321, 18.7514) (43.625, 18.8196) knots 0 0 0 1 1 1
  spline S236 degree 2 poles (43.625, 18.8196) (43.5725, 18.7098) (43.5724, 18.6261) knots 0 0 0 1 1 1
  spline S237 degree 2 poles (43.5724, 18.6261) (43.5722, 18.5136) (43.6387, 18.4181) knots 0 0 0 1 1 1
  spline S238 degree 2 poles (43.6387, 18.4181) (43.7053, 18.3225) (43.8111, 18.253) knots 0 0 0 1 1 1
  spline S239 degree 2 poles (43.8111, 18.253) (43.9169, 18.1835) (44.0516, 18.1454) knots 0 0 0 1 1 1
  spline S240 degree 2 poles (44.0516, 18.1454) (44.1862, 18.1073) (44.3196, 18.1071) knots 0 0 0 1 1 1
  line L85 (44.3196, 18.1071) -> (44.351, 18.107)
  line L86 (44.351, 18.107) -> (44.3544, 20.325)
  line L87 (44.3544, 20.325) -> (44.4562, 20.2385)
  spline S241 degree 2 poles (44.4562, 20.2385) (44.5447, 19.9533) (44.6765, 19.7334) knots 0 0 0 1 1 1
  spline S242 degree 2 poles (44.6765, 19.7334) (44.8082, 19.5135) (44.9702, 19.3576) knots 0 0 0 1 1 1
  spline S243 degree 2 poles (44.9702, 19.3576) (45.1321, 19.2018) (45.3216, 19.1099) knots 0 0 0 1 1 1
  spline S244 degree 2 poles (45.3216, 19.1099) (45.5111, 19.0181) (45.7176, 18.989) knots 0 0 0 1 1 1
  line L88 (45.7176, 18.989) -> (45.9656, 18.646)
  line L89 (45.9656, 18.646) -> (44.5598, 17.7903)
  line L90 (44.5598, 17.7903) -> (44.5595, 17.6019)
  line L91 (44.5595, 17.6019) -> (46.0294, 17.5997)
  line L92 (46.0294, 17.5997) -> (46.173, 17.4033)
  line L93 (46.173, 17.4033) -> (42.9977, 17.4081)
  line L94 (42.9977, 17.4081) -> (42.8542, 17.6045)
  line L95 (44.5603, 18.1381) -> (45.4923, 18.7095)
  spline S245 degree 2 poles (45.4923, 18.7095) (45.372, 18.7594) (45.2492, 18.8393) knots 0 0 0 1 1 1
  spline S246 degree 2 poles (45.2492, 18.8393) (45.1264, 18.9193) (45.0063, 19.0319) knots 0 0 0 1 1 1
  spline S247 degree 2 poles (45.0063, 19.0319) (44.8861, 19.1446) (44.7739, 19.2925) knots 0 0 0 1 1 1
  spline S248 degree 2 poles (44.7739, 19.2925) (44.6617, 19.4405) (44.5625, 19.6237) knots 0 0 0 1 1 1
  line L96 (44.5625, 19.6237) -> (44.5603, 18.1381)
  line L97 (40.8298, 17.6076) -> (41.3659, 17.6068)
  line L98 (41.3659, 17.6068) -> (41.3701, 20.3295)
  line L99 (41.3701, 20.3295) -> (41.4719, 20.2326)
  spline S249 degree 2 poles (41.4719, 20.2326) (41.5526, 19.9474) (41.6765, 19.734) knots 0 0 0 1 1 1
  spline S250 degree 2 poles (41.6765, 19.734) (41.8004, 19.5207) (41.9571, 19.3635) knots 0 0 0 1 1 1
  spline S251 degree 2 poles (41.9571, 19.3635) (42.1138, 19.2063) (42.3059, 19.1171) knots 0 0 0 1 1 1
  spline S252 degree 2 poles (42.3059, 19.1171) (42.498, 19.0279) (42.7281, 18.9988) knots 0 0 0 1 1 1
  line L100 (42.7281, 18.9988) -> (42.9734, 18.6505)
  line L101 (42.9734, 18.6505) -> (41.5755, 17.7895)
  line L102 (41.5755, 17.7895) -> (41.5752, 17.6064)
  line L103 (41.5752, 17.6064) -> (43.0373, 17.6042)
  line L104 (43.0373, 17.6042) -> (43.1808, 17.4079)
  line L105 (43.1808, 17.4079) -> (40.9733, 17.4112)
  line L106 (40.9733, 17.4112) -> (40.8298, 17.6076)
  line L107 (41.576, 18.1269) -> (42.508, 18.6983)
  spline S253 degree 2 poles (42.508, 18.6983) (42.3433, 18.7901) (42.2114, 18.8832) knots 0 0 0 1 1 1
  spline S254 degree 2 poles (42.2114, 18.8832) (42.0794, 18.9762) (41.9697, 19.0823) knots 0 0 0 1 1 1
  spline S255 degree 2 poles (41.9697, 19.0823) (41.86, 19.1884) (41.7648, 19.3154) knots 0 0 0 1 1 1
  spline S256 degree 2 poles (41.7648, 19.3154) (41.6695, 19.4424) (41.5782, 19.6047) knots 0 0 0 1 1 1
  line L108 (41.5782, 19.6047) -> (41.576, 18.1269)
  spline S257 degree 2 poles (42.0939, 19.9047) (42.0941, 20.0146) (42.1687, 20.089) knots 0 0 0 1 1 1
  spline S258 degree 2 poles (42.1687, 20.089) (42.2434, 20.1634) (42.3532, 20.1632) knots 0 0 0 1 1 1
  spline S259 degree 2 poles (42.3532, 20.1632) (42.4631, 20.1631) (42.5375, 20.0884) knots 0 0 0 1 1 1
  spline S260 degree 2 poles (42.5375, 20.0884) (42.6119, 20.0138) (42.6118, 19.9039) knots 0 0 0 1 1 1
  spline S261 degree 2 poles (42.6118, 19.9039) (42.6116, 19.7941) (42.537, 19.7196) knots 0 0 0 1 1 1
  spline S262 degree 2 poles (42.537, 19.7196) (42.4623, 19.6452) (42.3525, 19.6454) knots 0 0 0 1 1 1
  spline S263 degree 2 poles (42.3525, 19.6454) (42.2426, 19.6455) (42.1682, 19.7202) knots 0 0 0 1 1 1
  spline S264 degree 2 poles (42.1682, 19.7202) (42.0937, 19.7948) (42.0939, 19.9047) knots 0 0 0 1 1 1
  line L109 (39.0774, 17.6102) -> (39.3572, 17.6098)
  spline S265 degree 2 poles (39.3572, 17.6098) (39.4828, 17.6096) (39.6215, 17.6669) knots 0 0 0 1 1 1
  spline S266 degree 2 poles (39.6215, 17.6669) (39.7602, 17.7243) (39.8924, 17.8261) knots 0 0 0 1 1 1
  spline S267 degree 2 poles (39.8924, 17.8261) (40.0247, 17.9279) (40.1439, 18.0689) knots 0 0 0 1 1 1
  spline S268 degree 2 poles (40.1439, 18.0689) (40.2631, 18.21) (40.3536, 18.3786) knots 0 0 0 1 1 1
  spline S269 degree 2 poles (40.3536, 18.3786) (40.4441, 18.5471) (40.498, 18.7367) knots 0 0 0 1 1 1
  spline S270 degree 2 poles (40.498, 18.7367) (40.5519, 18.9262) (40.5522, 19.125) knots 0 0 0 1 1 1
  spline S271 degree 2 poles (40.5522, 19.125) (40.5525, 19.3185) (40.5135, 19.4768) knots 0 0 0 1 1 1
  spline S272 degree 2 poles (40.5135, 19.4768) (40.4745, 19.6351) (40.4067, 19.7516) knots 0 0 0 1 1 1
  spline S273 degree 2 poles (40.4067, 19.7516) (40.3388, 19.8681) (40.2461, 19.9389) knots 0 0 0 1 1 1
  spline S274 degree 2 poles (40.2461, 19.9389) (40.1534, 20.0096) (40.0461, 20.0307) knots 0 0 0 1 1 1
  spline S275 degree 2 poles (40.0461, 20.0307) (40.0487, 20.0124) (40.05, 19.9967) knots 0 0 0 1 1 1
  spline S276 degree 2 poles (40.05, 19.9967) (40.0513, 19.981) (40.0513, 19.9653) knots 0 0 0 1 1 1
  spline S277 degree 2 poles (40.0513, 19.9653) (40.0511, 19.8685) (40.0197, 19.8084) knots 0 0 0 1 1 1
  spline S278 degree 2 poles (40.0197, 19.8084) (39.9882, 19.7483) (39.9384, 19.7157) knots 0 0 0 1 1 1
  spline S279 degree 2 poles (39.9384, 19.7157) (39.8887, 19.6831) (39.8324, 19.6727) knots 0 0 0 1 1 1
  spline S280 degree 2 poles (39.8324, 19.6727) (39.7762, 19.6623) (39.7239, 19.6624) knots 0 0 0 1 1 1
  spline S281 degree 2 poles (39.7239, 19.6624) (39.6611, 19.6625) (39.6036, 19.6874) knots 0 0 0 1 1 1
  spline S282 degree 2 poles (39.6036, 19.6874) (39.5461, 19.7124) (39.503, 19.7582) knots 0 0 0 1 1 1
  spline S283 degree 2 poles (39.503, 19.7582) (39.4599, 19.8041) (39.4339, 19.8656) knots 0 0 0 1 1 1
  spline S284 degree 2 poles (39.4339, 19.8656) (39.4078, 19.9271) (39.4079, 20.0003) knots 0 0 0 1 1 1
  spline S285 degree 2 poles (39.4079, 20.0003) (39.408, 20.0657) (39.433, 20.1297) knots 0 0 0 1 1 1
  spline S286 degree 2 poles (39.433, 20.1297) (39.4579, 20.1938) (39.5064, 20.2447) knots 0 0 0 1 1 1
  spline S287 degree 2 poles (39.5064, 20.2447) (39.5548, 20.2956) (39.6268, 20.3269) knots 0 0 0 1 1 1
  spline S288 degree 2 poles (39.6268, 20.3269) (39.6988, 20.3582) (39.7929, 20.358) knots 0 0 0 1 1 1
  spline S289 degree 2 poles (39.7929, 20.358) (39.9106, 20.3579) (40.0191, 20.3211) knots 0 0 0 1 1 1
  spline S290 degree 2 poles (40.0191, 20.3211) (40.1276, 20.2843) (40.2191, 20.2227) knots 0 0 0 1 1 1
  spline S291 degree 2 poles (40.2191, 20.2227) (40.3105, 20.1611) (40.3862, 20.0799) knots 0 0 0 1 1 1
  spline S292 degree 2 poles (40.3862, 20.0799) (40.462, 19.9987) (40.5168, 19.9071) knots 0 0 0 1 1 1
  spline S293 degree 2 poles (40.5168, 19.9071) (40.5559, 19.8416) (40.5976, 19.7487) knots 0 0 0 1 1 1
  spline S294 degree 2 poles (40.5976, 19.7487) (40.6393, 19.6558) (40.6718, 19.5315) knots 0 0 0 1 1 1
  spline S295 degree 2 poles (40.6718, 19.5315) (40.7043, 19.4072) (40.725, 19.2516) knots 0 0 0 1 1 1
  spline S296 degree 2 poles (40.725, 19.2516) (40.7457, 19.0959) (40.7454, 18.8998) knots 0 0 0 1 1 1
  spline S297 degree 2 poles (40.7454, 18.8998) (40.7451, 18.6905) (40.6977, 18.4983) knots 0 0 0 1 1 1
  spline S298 degree 2 poles (40.6977, 18.4983) (40.6503, 18.3062) (40.5716, 18.1402) knots 0 0 0 1 1 1
  spline S299 degree 2 poles (40.5716, 18.1402) (40.4929, 17.9742) (40.3894, 17.8384) knots 0 0 0 1 1 1
  spline S300 degree 2 poles (40.3894, 17.8384) (40.2859, 17.7025) (40.1759, 17.6085) knots 0 0 0 1 1 1
  line L110 (40.1759, 17.6085) -> (41.0128, 17.6073)
  line L111 (41.0128, 17.6073) -> (41.1564, 17.4109)
  line L112 (41.1564, 17.4109) -> (39.2209, 17.4138)
  line L113 (39.2209, 17.4138) -> (39.0774, 17.6102)
  line L114 (37.053, 17.6133) -> (37.5891, 17.6125)
  line L115 (37.5891, 17.6125) -> (37.5932, 20.3352)
  line L116 (37.5932, 20.3352) -> (37.6951, 20.2383)
  spline S301 degree 2 poles (37.6951, 20.2383) (37.7758, 19.9531) (37.8997, 19.7397) knots 0 0 0 1 1 1
  spline S302 degree 2 poles (37.8997, 19.7397) (38.0236, 19.5264) (38.1803, 19.3692) knots 0 0 0 1 1 1
  spline S303 degree 2 poles (38.1803, 19.3692) (38.337, 19.212) (38.5291, 19.1228) knots 0 0 0 1 1 1
  spline S304 degree 2 poles (38.5291, 19.1228) (38.7212, 19.0336) (38.9513, 19.0045) knots 0 0 0 1 1 1
  line L117 (38.9513, 19.0045) -> (39.1966, 18.6562)
  line L118 (39.1966, 18.6562) -> (37.7987, 17.7952)
  line L119 (37.7987, 17.7952) -> (37.7984, 17.6121)
  line L120 (37.7984, 17.6121) -> (39.2605, 17.6099)
  line L121 (39.2605, 17.6099) -> (39.404, 17.4136)
  line L122 (39.404, 17.4136) -> (37.1965, 17.4169)
  line L123 (37.1965, 17.4169) -> (37.053, 17.6133)
  line L124 (37.7992, 18.1326) -> (38.7312, 18.704)
  spline S305 degree 2 poles (38.7312, 18.704) (38.5665, 18.7958) (38.4346, 18.8889) knots 0 0 0 1 1 1
  spline S306 degree 2 poles (38.4346, 18.8889) (38.3026, 18.9819) (38.1929, 19.088) knots 0 0 0 1 1 1
  spline S307 degree 2 poles (38.1929, 19.088) (38.0832, 19.1941) (37.988, 19.3211) knots 0 0 0 1 1 1
  spline S308 degree 2 poles (37.988, 19.3211) (37.8927, 19.4481) (37.8014, 19.6104) knots 0 0 0 1 1 1
  line L125 (37.8014, 19.6104) -> (37.7992, 18.1326)
  line L126 (34.8036, 17.6167) -> (35.3398, 17.6158)
  line L127 (35.3398, 17.6158) -> (35.3439, 20.3334)
  line L128 (35.3439, 20.3334) -> (35.4457, 20.226)
  spline S309 degree 2 poles (35.4457, 20.226) (35.4455, 20.0507) (35.4858, 19.8781) knots 0 0 0 1 1 1
  spline S310 degree 2 poles (35.4858, 19.8781) (35.526, 19.7054) (35.5951, 19.5483) knots 0 0 0 1 1 1
  spline S311 degree 2 poles (35.5951, 19.5483) (35.6642, 19.3913) (35.7581, 19.2565) knots 0 0 0 1 1 1
  spline S312 degree 2 poles (35.7581, 19.2565) (35.8521, 19.1216) (35.9605, 19.0221) knots 0 0 0 1 1 1
  spline S313 degree 2 poles (35.9605, 19.0221) (36.0689, 18.9225) (36.1878, 18.8661) knots 0 0 0 1 1 1
  spline S314 degree 2 poles (36.1878, 18.8661) (36.3067, 18.8097) (36.4244, 18.8095) knots 0 0 0 1 1 1
  spline S315 degree 2 poles (36.4244, 18.8095) (36.3514, 18.9456) (36.3516, 19.0659) knots 0 0 0 1 1 1
  spline S316 degree 2 poles (36.3516, 19.0659) (36.3517, 19.1549) (36.3871, 19.2267) knots 0 0 0 1 1 1
  spline S317 degree 2 poles (36.3871, 19.2267) (36.4225, 19.2986) (36.4789, 19.3482) knots 0 0 0 1 1 1
  spline S318 degree 2 poles (36.4789, 19.3482) (36.5352, 19.3978) (36.6045, 19.4252) knots 0 0 0 1 1 1
  spline S319 degree 2 poles (36.6045, 19.4252) (36.6739, 19.4525) (36.7393, 19.4524) knots 0 0 0 1 1 1
  spline S320 degree 2 poles (36.7393, 19.4524) (36.8386, 19.4523) (36.9184, 19.4156) knots 0 0 0 1 1 1
  spline S321 degree 2 poles (36.9184, 19.4156) (36.9981, 19.3788) (37.0555, 19.316) knots 0 0 0 1 1 1
  spline S322 degree 2 poles (37.0555, 19.316) (37.113, 19.2531) (37.1429, 19.1707) knots 0 0 0 1 1 1
  spline S323 degree 2 poles (37.1429, 19.1707) (37.1729, 19.0882) (37.1727, 18.9967) knots 0 0 0 1 1 1
  spline S324 degree 2 poles (37.1727, 18.9967) (37.1726, 18.8711) (37.1227, 18.7744) knots 0 0 0 1 1 1
  spline S325 degree 2 poles (37.1227, 18.7744) (37.0729, 18.6778) (36.9878, 18.6125) knots 0 0 0 1 1 1
  spline S326 degree 2 poles (36.9878, 18.6125) (36.9027, 18.5472) (36.7901, 18.5147) knots 0 0 0 1 1 1
  spline S327 degree 2 poles (36.7901, 18.5147) (36.6776, 18.4822) (36.5521, 18.4824) knots 0 0 0 1 1 1
  spline S328 degree 2 poles (36.5521, 18.4824) (36.4501, 18.4825) (36.3168, 18.522) knots 0 0 0 1 1 1
  spline S329 degree 2 poles (36.3168, 18.522) (36.1834, 18.5614) (36.0462, 18.6558) knots 0 0 0 1 1 1
  spline S330 degree 2 poles (36.0462, 18.6558) (35.9091, 18.7501) (35.7785, 18.9046) knots 0 0 0 1 1 1
  spline S331 degree 2 poles (35.7785, 18.9046) (35.648, 19.0592) (35.5516, 19.2868) knots 0 0 0 1 1 1
  line L129 (35.5516, 19.2868) -> (35.549, 17.6155)
  line L130 (35.549, 17.6155) -> (37.236, 17.613)
  line L131 (37.236, 17.613) -> (37.3796, 17.4166)
  line L132 (37.3796, 17.4166) -> (34.9472, 17.4203)
  line L133 (34.9472, 17.4203) -> (34.8036, 17.6167)
  line L134 (31.4479, 17.6217) -> (31.9841, 17.6209)
  line L135 (31.9841, 17.6209) -> (31.9882, 20.3384)
  line L136 (31.9882, 20.3384) -> (32.09, 20.231)
  spline S332 degree 2 poles (32.09, 20.231) (32.0898, 20.0558) (32.13, 19.8831) knots 0 0 0 1 1 1
  spline S333 degree 2 poles (32.13, 19.8831) (32.1703, 19.7104) (32.2394, 19.5534) knots 0 0 0 1 1 1
  spline S334 degree 2 poles (32.2394, 19.5534) (32.3085, 19.3964) (32.4024, 19.2615) knots 0 0 0 1 1 1
  spline S335 degree 2 poles (32.4024, 19.2615) (32.4964, 19.1267) (32.6048, 19.0271) knots 0 0 0 1 1 1
  spline S336 degree 2 poles (32.6048, 19.0271) (32.7132, 18.9276) (32.8321, 18.8712) knots 0 0 0 1 1 1
  spline S337 degree 2 poles (32.8321, 18.8712) (32.951, 18.8147) (33.0687, 18.8146) knots 0 0 0 1 1 1
  spline S338 degree 2 poles (33.0687, 18.8146) (32.9957, 18.9507) (32.9959, 19.071) knots 0 0 0 1 1 1
  spline S339 degree 2 poles (32.9959, 19.071) (32.996, 19.1599) (33.0314, 19.2318) knots 0 0 0 1 1 1
  spline S340 degree 2 poles (33.0314, 19.2318) (33.0668, 19.3037) (33.1231, 19.3533) knots 0 0 0 1 1 1
  spline S341 degree 2 poles (33.1231, 19.3533) (33.1795, 19.4029) (33.2488, 19.4303) knots 0 0 0 1 1 1
  spline S342 degree 2 poles (33.2488, 19.4303) (33.3182, 19.4576) (33.3835, 19.4575) knots 0 0 0 1 1 1
  spline S343 degree 2 poles (33.3835, 19.4575) (33.4829, 19.4574) (33.5627, 19.4206) knots 0 0 0 1 1 1
  spline S344 degree 2 poles (33.5627, 19.4206) (33.6424, 19.3839) (33.6998, 19.321) knots 0 0 0 1 1 1
  spline S345 degree 2 poles (33.6998, 19.321) (33.7573, 19.2582) (33.7872, 19.1757) knots 0 0 0 1 1 1
  spline S346 degree 2 poles (33.7872, 19.1757) (33.8172, 19.0933) (33.817, 19.0018) knots 0 0 0 1 1 1
  spline S347 degree 2 poles (33.817, 19.0018) (33.8168, 18.8762) (33.767, 18.7795) knots 0 0 0 1 1 1
  spline S348 degree 2 poles (33.767, 18.7795) (33.7172, 18.6828) (33.6321, 18.6176) knots 0 0 0 1 1 1
  spline S349 degree 2 poles (33.6321, 18.6176) (33.547, 18.5523) (33.4344, 18.5198) knots 0 0 0 1 1 1
  spline S350 degree 2 poles (33.4344, 18.5198) (33.3219, 18.4872) (33.1964, 18.4874) knots 0 0 0 1 1 1
  spline S351 degree 2 poles (33.1964, 18.4874) (33.0944, 18.4876) (32.961, 18.527) knots 0 0 0 1 1 1
  spline S352 degree 2 poles (32.961, 18.527) (32.8277, 18.5665) (32.6905, 18.6608) knots 0 0 0 1 1 1
  spline S353 degree 2 poles (32.6905, 18.6608) (32.5534, 18.7552) (32.4228, 18.9097) knots 0 0 0 1 1 1
  spline S354 degree 2 poles (32.4228, 18.9097) (32.2923, 19.0642) (32.1959, 19.2919) knots 0 0 0 1 1 1
  line L137 (32.1959, 19.2919) -> (32.1933, 17.6206)
  line L138 (32.1933, 17.6206) -> (33.8803, 17.6181)
  line L139 (33.8803, 17.6181) -> (34.0239, 17.4217)
  line L140 (34.0239, 17.4217) -> (31.5915, 17.4253)
  line L141 (31.5915, 17.4253) -> (31.4479, 17.6217)
  line L142 (30.488, 17.6232) -> (31.0242, 17.6224)
  line L143 (31.0242, 17.6224) -> (31.0283, 20.366)
  line L144 (31.0283, 20.366) -> (31.2373, 20.1774)
  line L145 (31.2373, 20.1774) -> (31.2341, 18.0667)
  spline S355 degree 2 poles (31.2341, 18.0667) (31.2341, 18.0327) (31.2679, 17.962) knots 0 0 0 1 1 1
  spline S356 degree 2 poles (31.2679, 17.962) (31.3018, 17.8913) (31.3501, 17.818) knots 0 0 0 1 1 1
  spline S357 degree 2 poles (31.3501, 17.818) (31.3984, 17.7447) (31.4545, 17.6871) knots 0 0 0 1 1 1
  spline S358 degree 2 poles (31.4545, 17.6871) (31.5107, 17.6295) (31.5551, 17.6216) knots 0 0 0 1 1 1
  line L146 (31.5551, 17.6216) -> (31.631, 17.6214)
  line L147 (31.631, 17.6214) -> (31.7745, 17.4251)
  line L148 (31.7745, 17.4251) -> (31.5862, 17.4253)
  spline S359 degree 2 poles (31.5862, 17.4253) (31.5209, 17.4411) (31.4738, 17.4687) knots 0 0 0 1 1 1
  spline S360 degree 2 poles (31.4738, 17.4687) (31.4268, 17.4962) (31.3876, 17.5381) knots 0 0 0 1 1 1
  spline S361 degree 2 poles (31.3876, 17.5381) (31.3485, 17.58) (31.3132, 17.6389) knots 0 0 0 1 1 1
  spline S362 degree 2 poles (31.3132, 17.6389) (31.278, 17.6978) (31.2337, 17.7764) knots 0 0 0 1 1 1
  line L149 (31.2337, 17.7764) -> (31.2324, 16.9159)
  spline S363 degree 2 poles (31.2324, 16.9159) (31.1827, 16.9395) (31.1501, 17.0049) knots 0 0 0 1 1 1
  spline S364 degree 2 poles (31.1501, 17.0049) (31.1175, 17.0703) (31.0954, 17.1488) knots 0 0 0 1 1 1
  spline S365 degree 2 poles (31.0954, 17.1488) (31.0733, 17.2273) (31.0577, 17.3032) knots 0 0 0 1 1 1
  spline S366 degree 2 poles (31.0577, 17.3032) (31.0421, 17.3791) (31.0265, 17.4262) knots 0 0 0 1 1 1
  line L150 (31.0265, 17.4262) -> (30.6316, 17.4268)
  line L151 (30.6316, 17.4268) -> (30.488, 17.6232)
  spline S367 degree 2 poles (50.2029, 44.0682) (49.9437, 44.0701) (49.6977, 44.2049) knots 0 0 0 1 1 1
  spline S368 degree 2 poles (49.6977, 44.2049) (49.4518, 44.3398) (49.3158, 44.5884) knots 0 0 0 1 1 1
  spline S369 degree 2 poles (49.3158, 44.5884) (49.1798, 44.837) (49.1818, 45.1057) knots 0 0 0 1 1 1
  spline S370 degree 2 poles (49.1818, 45.1057) (49.1838, 45.3718) (49.3213, 45.6163) knots 0 0 0 1 1 1
  spline S371 degree 2 poles (49.3213, 45.6163) (49.4589, 45.8609) (49.7047, 45.9948) knots 0 0 0 1 1 1
  spline S372 degree 2 poles (49.7047, 45.9948) (49.9506, 46.1288) (50.218, 46.1268) knots 0 0 0 1 1 1
  spline S373 degree 2 poles (50.218, 46.1268) (50.4854, 46.1248) (50.7293, 45.9873) knots 0 0 0 1 1 1
  spline S374 degree 2 poles (50.7293, 45.9873) (50.9731, 45.8498) (51.1078, 45.6032) knots 0 0 0 1 1 1
  spline S375 degree 2 poles (51.1078, 45.6032) (51.2424, 45.3566) (51.2404, 45.0906) knots 0 0 0 1 1 1
  spline S376 degree 2 poles (51.2404, 45.0906) (51.2384, 44.8219) (51.0982, 44.5753) knots 0 0 0 1 1 1
  spline S377 degree 2 poles (51.0982, 44.5753) (50.9579, 44.3287) (50.71, 44.1975) knots 0 0 0 1 1 1
  spline S378 degree 2 poles (50.71, 44.1975) (50.4621, 44.0663) (50.2029, 44.0682) knots 0 0 0 1 1 1
  spline S379 degree 2 poles (50.2041, 44.2387) (50.421, 44.2371) (50.6272, 44.3468) knots 0 0 0 1 1 1
  spline S380 degree 2 poles (50.6272, 44.3468) (50.8333, 44.4565) (50.9508, 44.6623) knots 0 0 0 1 1 1
  spline S381 degree 2 poles (50.9508, 44.6623) (51.0682, 44.8681) (51.0699, 45.0919) knots 0 0 0 1 1 1
  spline S382 degree 2 poles (51.0699, 45.0919) (51.0715, 45.3142) (50.9591, 45.519) knots 0 0 0 1 1 1
  spline S383 degree 2 poles (50.9591, 45.519) (50.8467, 45.7238) (50.6429, 45.8392) knots 0 0 0 1 1 1
  spline S384 degree 2 poles (50.6429, 45.8392) (50.4391, 45.9546) (50.2167, 45.9563) knots 0 0 0 1 1 1
  spline S385 degree 2 poles (50.2167, 45.9563) (49.9944, 45.9579) (49.7889, 45.8455) knots 0 0 0 1 1 1
  spline S386 degree 2 poles (49.7889, 45.8455) (49.5834, 45.7331) (49.4687, 45.53) knots 0 0 0 1 1 1
  spline S387 degree 2 poles (49.4687, 45.53) (49.354, 45.3269) (49.3523, 45.1045) knots 0 0 0 1 1 1
  spline S388 degree 2 poles (49.3523, 45.1045) (49.3507, 44.8808) (49.4645, 44.6732) knots 0 0 0 1 1 1
  spline S389 degree 2 poles (49.4645, 44.6732) (49.5782, 44.4657) (49.7834, 44.353) knots 0 0 0 1 1 1
  spline S390 degree 2 poles (49.7834, 44.353) (49.9886, 44.2403) (50.2041, 44.2387) knots 0 0 0 1 1 1
  line L152 (49.8815, 45.267) -> (49.7141, 45.3174)